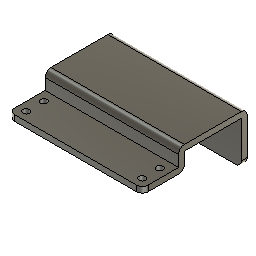
project (Autodesk Fusion 360 design; units mm, degrees)
Autodesk Fusion 360 part; units mm, degrees
note: some values were not read from the file. Set by a fixed rule: which sketch regions a step uses.
sketch "Sketch5" plane through (0, 0, 0) normal (0, 0, 1) x (1, 0, 0)
  line L0 (-40, 6) -> (40, 6) construction
  line L1 (40, 6) -> (40, 18) construction
  line L2 (40, 18) -> (-40, 18) construction
  line L3 (-40, 18) -> (-40, 6) construction
  circle A0 centre (-40, 18) radius 2.25
  circle A1 centre (-40, 6) radius 2.25
  circle A2 centre (40, 18) radius 2.25
  circle A3 centre (40, 6) radius 2.25
  line L4 (46, 24) -> (-46, 24)
  line L5 (-46, 24) -> (-46, 0)
  line L6 (-46, 0) -> (46, 0)
  line L7 (46, 0) -> (46, 24)
  line L8 (46, 24) -> (46, 25)
  line L9 (46, 25) -> (-46, 25)
  line L10 (-46, 25) -> (-46, 24)
  dimension "d20" = 80
  dimension "d21" = 12
  dimension "d22" = 4.5
  dimension "d42" = 6
  dimension "d56" = 92
  dimension "d70" = 1
  dimension "d71" = 25
  constraint horizontal L0
  constraint vertical L1
  constraint horizontal L2
  constraint vertical L3
  constraint coincident L2.end L3.start
  constraint coincident L0.start L3.end
  constraint coincident L1.end L2.start
  constraint coincident L0.end L1.start
  constraint equal A0 A2
  constraint equal A1 A3
  constraint equal A0 A1
  constraint midpoint origin L6
  constraint vertical L8
  constraint horizontal L9
  constraint vertical L10
  measures "d20" distance of L1.end L2.end
  measures "d21" distance of L0.start L2.end
  measures "d22" diameter of A0
  measures "d56" distance of L5.end L6.end
  measures "d70" distance of L4 L9
  measures "d71" distance of L6 L9
extrude "Extrude6" add sketch "Sketch5" against normal blind 4
sketch "Sketch9" plane through (0, 0, 0) normal (1, 0, 0) x (0, 1, 0)
  line L0 (25, -4) -> (29, -4)
  line L1 (29, -4) -> (29, 7.75)
  line L2 (29, 7.75) -> (68.3, 7.75)
  line L3 (68.3, 7.75) -> (68.3, -21.75)
  line L4 (68.3, -21.75) -> (72.3, -21.75)
  line L5 (72.3, -21.75) -> (72.3, 11.75)
  line L6 (72.3, 11.75) -> (25, 11.75)
  line L7 (25, 11.75) -> (25, 0)
  line L8 (25, 0) -> (29, 0) construction
  line L9 (48.65, 7.75) -> (48.65, 11.75) construction
  line L10 (25, 0) -> (25, -4)
  line L11 (25, -4) -> (25, 0)
  line L12 (0, 0) -> (25, 0)
  line L13 (25, 0) -> (25, -4)
  line L14 (25, -4) -> (0, -4)
  line L15 (0, -4) -> (0, 0)
  point P0 (68.3, -7)
  dimension "d52" = 7
  dimension "d53" = 14.75
  dimension "d55" = 14.75
  dimension "d72" = 72.3
  constraint coincident L1 L8.end
  constraint vertical L7
  constraint vertical L1
  constraint horizontal L6
  constraint horizontal L2
  constraint vertical L5
  constraint vertical L3
  constraint horizontal L4
  constraint horizontal L0
  constraint horizontal L8
  constraint midpoint L2 L9.start
  constraint midpoint L6 L9.end
  constraint vertical L9
  constraint coincident L3 P0
  constraint coincident L0.start L10.end
  constraint coincident L7.end L8.start
  constraint equal L8 L9
  constraint equal L8 L11
  measures "d52" vertical distance of L12.start P0
  measures "d53" distance of L4 P0
  measures "d55" distance of L2 P0
  measures "d72" distance of L12.start L5
extrude "Extrude7" add sketch "Sketch9" along normal mid plane 92 contours L0 L1 L2 L3 L4 L5 L6 L7 L10 L11 L13
fillet "Fillet3" radius 4 7 edges at (46, 70.3, -21.75) (-46, 70.3, -21.75) (0, 72.3, 11.75) (0, 25, 11.75) (0, 29, -4) (-46, 0, -2) (46, 0, -2)
sketch "Sketch10" plane through (0, 0, 0) normal (0, 1, 0) x (1, 0, 0)
  line L0 (15, 2) -> (15, 12) construction
  arc A0 (18.25, 11.9963) -> (11.75, 12) centre (15, 12) ccw
  arc A1 (11.75, 2.0001) -> (18.25, 2) centre (15, 2) ccw
  line L1 (11.75, 12) -> (11.75, 2.0001)
  line L2 (18.25, 2) -> (18.25, 11.9963)
  line L3 (15, 7) -> (0, 7) construction
  point P0 (0, 7)
  dimension "d63" = 10
  dimension "d64" = 3.25
  dimension "d68" = 15
  constraint vertical L0
  constraint coincident L0.end A0.centre
  constraint coincident L0.start A1.centre
  constraint parallel L0 L2
  constraint parallel L0 L1
  constraint tangent A0 L1
  constraint tangent A1 L2
  constraint midpoint L0 L3.start
  constraint coincident P0 L3.end
  constraint horizontal L3
  measures "d63" distance of L0.start L0.end
  measures "d64" radius of A0
  measures "d68" distance of L3.start P0
extrude "Extrude8" cut sketch "Sketch10" along normal through all from surface at 68.3
equation "Thickness = 4 mm"
equation "d47 = -Thickness"
equation "d52 = ( MountHoleSpacing - 148 mm ) / 2"
equation "d53 = ( ( MountHoleTolerance + MountHoleSize ) / 2 ) + MountHoleSize"
equation "d55 = d53"
equation "d57 = d56"
equation "d60 = Thickness"
equation "MountHoleSpacing = 162 mm"
equation "MountHoleTolerance = 10 mm"
equation "d63 = MountHoleTolerance"
equation "d64 = ( 6.5 / 2 ) * 1 mm"
equation "MountHoleSize = 6.5 mm"
equation "SurfaceOffset = 30 mm"
equation "d72 = 42.3 mm + SurfaceOffset"
